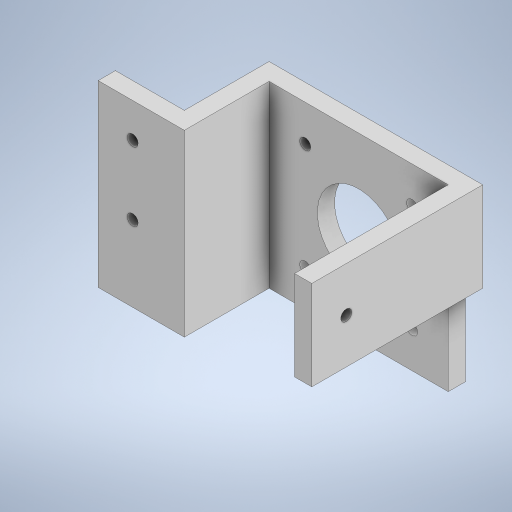
# Autodesk Inventor part: Motor Mount
Saved by Autodesk Inventor 2023.1 (Build 271208000, 208)
## iProperties
Created: 2022-10-30
Part Number: Motor Mount
Material: Generic
Document SubType Name: Modeling
Designer: nicol
Density: 1 g/cm^3
Appearance: Default
Author: nicol
Autodesk Inventor part; units mm, degrees
ref_plane "YZ Plane" through (0, 0, 0) normal (1, 0, 0) x (0, 1, 0)
ref_plane "XZ Plane" through (0, 0, 0) normal (0, 1, 0) x (-1, 0, 0)
ref_plane "XY Plane" through (0, 0, 0) normal (0, 0, 1) x (1, 0, 0)
sketch "Sketch1" plane through (0, 0, 0) normal (0, 0, 1) x (1, 0, 0)
  line L0 (0, 0) -> (52, 0)
  line L1 (52, 0) -> (52, 52)
  line L2 (52, 52) -> (0, 52)
  line L3 (0, 52) -> (0, 0)
  line L4 (0, 0) -> (5, 0)
  line L5 (52, 0) -> (45, 0)
  line L6 (10.5, 41.5) -> (41.5, 41.5) construction
  line L7 (41.5, 41.5) -> (41.5, 10.5) construction
  line L8 (41.5, 10.5) -> (10.5, 10.5) construction
  line L9 (10.5, 10.5) -> (10.5, 41.5) construction
  circle A0 centre (26, 26) radius 12
  line L10 (5, 47) -> (47, 47)
  line L11 (47, 47) -> (47, 5)
  line L12 (47, 5) -> (5, 5)
  line L13 (5, 5) -> (5, 47)
  line L14 (52, 52) -> (57, 52)
  line L15 (57, 52) -> (57, 26)
  line L16 (57, 26) -> (52, 26)
  line L17 (52, 26) -> (52, 52)
  line L18 (0, 52) -> (-5, 52)
  line L19 (-5, 52) -> (-5, 0)
  line L20 (-5, 0) -> (0, 0)
  line L21 (0, 0) -> (0, 52)
  point P0 (41.5, 26)
  point P1 (47, 26)
  point P2 (26, 41.5)
  point P3 (26, 47)
  point P4 (26, 52)
  dimension "d0" = 31
  dimension "d1" = 42
  dimension "d5" = 5
  dimension "d6" = 5
  dimension "d7" = 24
  dimension "d32" = 5
  dimension "d37" = 5
  constraints: 44 end point, 10 parallel, 8 perpendicular, 7 horizontal, 6 midpoint, 4 coincident, 3 vertical alignment, 2 horizontal alignment, 1 centre point, 1 collinear
  measures "d0" distance of L7.end L8.end
  measures "d1" distance of L10.end L11.end
  measures "d5" distance between parallel lines of L0 L12
  measures "d6" distance between parallel lines of L2 L10
  measures "d7" diameter of A0
  measures "d32" distance of L15.end L16.end
  measures "d37" distance of L2.end L18.end
extrude "Extrusion1" add sketch "Sketch1" against normal blind 5 contours L3 L2 L1 L0
extrude "Extrusion2" add sketch "Sketch1" against normal blind 5 contours L10 L11 L12 L13
extrude "Extrusion4" add sketch "Sketch1" along normal blind 44.6 and the other way blind 5 contours L14 L15 L16 L1
extrude "Extrusion5" add sketch "Sketch1" along normal blind 24.6 and the other way blind 5 contours L20 L19 L18 L3
hole "Hole1" at (10.5, 41.5, 0) at (41.5, 41.5, 0) at (41.5, 10.5, 0) at (10.5, 10.5, 0) direction (0, 0, -1) diameter 3.2 end through all
sketch "Sketch4" plane through (52, 52, 44.6) normal (0, 1, 0) x (1, 0, 0)
  line L0 (-57, 20) -> (-77, 20)
  line L1 (-77, 20) -> (-77, 25)
  line L2 (-77, 25) -> (-57, 25)
  line L3 (-57, 25) -> (-57, 20)
  point P0 (-52, 44.6)
  dimension "d42" = 20
  dimension "d43" = 5
  constraints: 8 end point, 2 parallel, 1 horizontal, 1 perpendicular
  measures "d42" distance of L1.end L2.end
  measures "d43" distance of L0.end L1.end
extrude "Extrusion6" add sketch "Sketch4" against normal up to surface (52 mm away)
sketch "Sketch5" plane through (57, 26, 44.6) normal (1, 0, 0) x (0, 0, -1)
  line L0 (0, 0) -> (0, 26) projected
  line L1 (0, 26) -> (49.6, 26) projected
  line L2 (49.6, 0) -> (0, 0) projected
  point P0 (44.6, -26)
  point P1 (10, 13)
  dimension "d46" = 10
  dimension "d47" = 13
  dimension "d48" = 13
  measures "d46" distance from line of L0 point (10, 13)
  measures "d47" distance from line of L1 point (10, 13)
  measures "d48" distance from line of L2 point (10, 13)
sketch "Sketch6" plane through (-5, 52, 19.6) normal (0, 0, -1) x (-1, 0, 0)
  line L0 (0, -52) -> (20, -52) projected
  line L1 (20, 0) -> (20, -52) projected
  line L2 (0, 0) -> (20, 0) projected
  line L3 (0, -52) -> (0, 0) projected
  point P0 (-5, -52)
  point P1 (10, -10)
  point P2 (10, -30)
  point P3 (10, -52)
  point P4 (10, 0)
  dimension "d49" = 10
  dimension "d65" = 20
  constraints: 3 vertical alignment, 2 midpoint
  measures "d49" distance from line of L2 point (10, -10)
  measures "d65" distance of point (10, -10) point (10, -30)
hole "Hole3" at (-15, 42, 19.6) at (-15, 22, 19.6) direction (0, 0, 1) diameter 3.2 end through all
hole "Hole4" at (57, 39, 34.6) direction (-1, 0, 0) diameter 3.2 end through all
equation "\"d6\" = d5"
equation "\"d47\" = d48"
body "Solid1"
